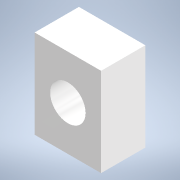
# Autodesk Inventor part: short back plate spacer
Saved by Autodesk Inventor 2022 (Build 260153000, 153)
## iProperties
Created: 2021-05-28
Part Number: short back plate spacer
Material: ABS Plastic
Document SubType Name: Modeling
Designer: benka
Density: 1.06 g/cm^3
Appearance: Smooth - White
Author: benka
Autodesk Inventor part; units mm, degrees
ref_plane "YZ Plane" through (0, 0, 0) normal (1, 0, 0) x (0, 1, 0)
ref_plane "XZ Plane" through (0, 0, 0) normal (0, 1, 0) x (-1, 0, 0)
ref_plane "XY Plane" through (0, 0, 0) normal (0, 0, 1) x (1, 0, 0)
sketch "Sketch1" plane through (0, 0, 0) normal (0, 0, 1) x (1, 0, 0)
  line L0 (-0.2511, -0.0105) -> (7.2489, -0.0105)
  line L1 (7.2489, -0.0105) -> (7.2489, 9.9895)
  line L2 (7.2489, 9.9895) -> (-0.2511, 9.9895)
  line L3 (-0.2511, 9.9895) -> (-0.2511, -0.0105)
  circle A0 centre (3.4989, 4.9895) radius 2
  point P0 (7.2471, -0.0105)
  dimension "d2" = 4
  dimension "d3" = 5
  dimension "d4" = 7.5
  dimension "d5" = 10
  dimension "d6" = 3.75
  constraints: 9 end point, 1 centre point, 1 horizontal, 1 vertical
  measures "d2" diameter of A0
  measures "d3" distance from line of L2 A0.centre
  measures "d4" distance between parallel lines of L1 L3
  measures "d5" distance between parallel lines of L0 L2
  measures "d6" distance from line of L3 A0.centre
extrude "Extrusion1" add sketch "Sketch1" along normal blind 5
body "Solid1"
